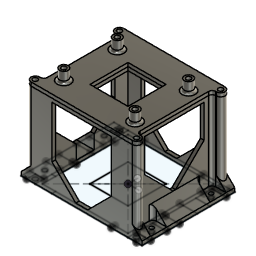
Battery Case (Autodesk Fusion 360 design; units mm, degrees)
Autodesk Fusion 360 part; units mm, degrees
sketch "Sketch1" plane through (0, 0, 0) normal (0, 0, 1) x (1, 0, 0)
  line L0 (36, 36) -> (-36, 36)
  line L1 (-36, 36) -> (-36, -36)
  line L2 (-36, -36) -> (36, -36)
  line L3 (36, -36) -> (36, 36)
  line L4 (36, 36) -> (-36, -36) construction
  line L5 (-36, 36) -> (36, -36) construction
  line L6 (-39, 39) -> (39, 39)
  line L7 (39, 39) -> (39, -39)
  line L8 (39, -39) -> (-39, -39)
  line L9 (-39, -39) -> (-39, 39)
  line L10 (-39, 39) -> (-50.8, 39)
  line L11 (-50.8, 39) -> (-50.8, -39)
  line L12 (-50.8, -39) -> (-39, -39)
  line L13 (39, -39) -> (50.8, -39)
  line L14 (50.8, -39) -> (50.8, 39)
  line L15 (50.8, 39) -> (39, 39)
  circle A0 centre (-45, 25) radius 1.7
  line L16 (0, 0) -> (0, 8)
  line L17 (0, 0) -> (9, 0)
  circle A1 centre (-45, -25) radius 1.7
  circle A2 centre (45, 25) radius 1.7
  circle A3 centre (45, -25) radius 1.7
  line L18 (-39, -25) -> (-36, -25)
  line L19 (39, -25) -> (36, -25)
  line L20 (-39, 25) -> (-36, 25)
  line L21 (39, 25) -> (36, 25)
  line L22 (-25, -39) -> (-25, -36)
  line L23 (25, -39) -> (25, -36)
  line L24 (-25, 39) -> (-25, 36)
  line L25 (25, 39) -> (25, 36)
  line L26 (-50.8, 31.8) -> (-39, 31.8)
  line L27 (50.8, 31.8) -> (39, 31.8)
  line L28 (-50.8, -31.8) -> (-39, -31.8)
  line L29 (50.8, -31.8) -> (39, -31.8)
  circle A4 centre (-42.6, 35.4) radius 2
  line L30 (-39, 31.8) -> (-46.2, 31.8)
  line L31 (-46.2, 31.8) -> (-46.2, 39)
  line L32 (-42.6, 35.4) -> (-39, 35.4)
  line L33 (-42.6, 35.4) -> (-42.6, 31.8)
  line L34 (-42.6, 35.4) -> (-46.2, 35.4)
  line L35 (-42.6, 35.4) -> (-42.6, 39)
  line L36 (39, 31.8) -> (46.2, 31.8)
  line L37 (46.2, 31.8) -> (46.2, 39)
  circle A5 centre (42.6, 35.4) radius 2
  line L38 (39, -31.8) -> (46.2, -31.8)
  line L39 (46.2, -31.8) -> (46.2, -39)
  circle A6 centre (42.6, -35.4) radius 2
  line L40 (-39, -31.8) -> (-46.2, -31.8)
  line L41 (-46.2, -31.8) -> (-46.2, -39)
  circle A7 centre (-42.6, -35.4) radius 2
  line L42 (-16, -16) -> (16, -16)
  line L43 (16, -16) -> (16, 16)
  line L44 (16, 16) -> (-16, 16)
  line L45 (-16, 16) -> (-16, -16)
  line L46 (-16, -16) -> (16, 16) construction
  line L47 (16, -16) -> (-16, 16) construction
  line L48 (-39, 7.5) -> (-36, 7.5)
  line L49 (39, 7.5) -> (36, 7.5)
  line L50 (-39, -7.5) -> (-36, -7.5)
  line L51 (39, -7.5) -> (36, -7.5)
  line L52 (39, 7.5) -> (50.8, 7.5)
  line L53 (50.8, 18.2) -> (39, 18.2)
  line L54 (-39, 7.5) -> (-50.8, 7.5)
  line L55 (-50.8, 18.2) -> (-39, 18.2)
  line L56 (39, -7.5) -> (50.8, -7.5)
  line L57 (50.8, -18.2) -> (39, -18.2)
  line L58 (-39, -7.5) -> (-50.8, -7.5)
  line L59 (-50.8, -18.2) -> (-39, -18.2)
  dimension "d1" = 72
  dimension "d2" = 72
  dimension "d3" = 3
  dimension "d4" = 3
  dimension "d5" = 3
  dimension "d6" = 3
  dimension "d7" = 101.6
  dimension "d8" = 50
  dimension "d9" = 90
  dimension "d10" = 3.4
  dimension "d13" = 50
  dimension "d14" = 50
  dimension "d20" = 7.2
  dimension "d24" = 4
  dimension "d25" = 7.2
  dimension "d27" = 7.2
  dimension "d34" = 20
  dimension "d37" = 15
  dimension "d38" = 6.8
  constraint horizontal L0
  constraint perpendicular L0 L1
  constraint parallel L0 L2
  constraint parallel L1 L3
  constraint coincident L4 L16.start
  constraint coincident L5 L16.start
  constraint coincident L16.start L17.start
  constraint horizontal L6
  constraint vertical L7
  constraint horizontal L8
  constraint vertical L9
  constraint perpendicular L9 L10
  constraint perpendicular L10 L11
  constraint perpendicular L14 L15
  constraint perpendicular L13 L14
  constraint perpendicular L7 L13
  constraint perpendicular L11 L12
  constraint equal L10 L15
  constraint vertical L16
  constraint perpendicular L16 L17
  constraint symmetric A0 L17 A1
  constraint symmetric A0 L16 A2
  constraint symmetric L16 A1 A3
  constraint coincident L9 L18.start
  constraint coincident L1 L18.end
  constraint perpendicular L1 L18
  constraint symmetric L16 L18.start L19.start
  constraint symmetric L16 L18.end L19.end
  constraint symmetric L17 L18.start L20.start
  constraint symmetric L17 L18.end L20.end
  constraint symmetric L17 L19.start L21.start
  constraint symmetric L17 L19.end L21.end
  constraint coincident L8 L22.start
  constraint coincident L2 L22.end
  constraint perpendicular L2 L22
  constraint symmetric L16 L22.start L23.start
  constraint symmetric L16 L22.end L23.end
  constraint symmetric L17 L22.start L24.start
  constraint symmetric L17 L22.end L24.end
  constraint symmetric L17 L23.start L25.start
  constraint symmetric L17 L23.end L25.end
  constraint coincident L11 L26.start
  constraint coincident L9 L26.end
  constraint perpendicular L9 L26
  constraint symmetric L16 L26.start L27.start
  constraint symmetric L16 L26.end L27.end
  constraint symmetric L17 L26.start L28.start
  constraint symmetric L17 L26.end L28.end
  constraint symmetric L17 L27.start L29.start
  constraint symmetric L17 L27.end L29.end
  constraint perpendicular L9 L30
  constraint coincident L10 L31.end
  constraint perpendicular L10 L31
  constraint coincident A4.centre L32.start
  constraint coincident L9 L32.end
  constraint perpendicular L9 L32
  constraint coincident L30 L33.end
  constraint perpendicular L30 L33
  constraint coincident L31 L34.end
  constraint perpendicular L31 L34
  constraint coincident L10 L35.end
  constraint perpendicular L10 L35
  constraint equal L32 L34
  constraint equal L33 L35
  constraint symmetric L16 A4 A5
  constraint symmetric L16 L30.end L36.end
  constraint symmetric L16 L31.end L37.end
  constraint symmetric L17 A4 A7
  constraint symmetric L17 L30.end L40.end
  constraint symmetric L17 L31.end L41.end
  constraint symmetric L17 L36.end L38.end
  constraint symmetric L17 L37.end L39.end
  constraint symmetric L17 A5 A6
  constraint horizontal L42
  constraint perpendicular L42 L43
  constraint parallel L42 L44
  constraint parallel L43 L45
  constraint coincident L46 L16.start
  constraint coincident L47 L16.start
  constraint coincident L4 L42.start
  constraint coincident L9 L48.start
  constraint coincident L1 L48.end
  constraint perpendicular L1 L48
  constraint symmetric L16 L48.start L49.start
  constraint symmetric L16 L48.end L49.end
  constraint symmetric L17 L48.start L50.start
  constraint symmetric L17 L48.end L50.end
  constraint symmetric L17 L49.start L51.start
  constraint symmetric L17 L49.end L51.end
  constraint coincident L14 L52.end
  constraint perpendicular L14 L52
  constraint coincident L14 L53.start
  constraint coincident L7 L53.end
  constraint perpendicular L7 L53
  constraint symmetric L16 L49.start L48.start
  constraint symmetric L16 L52.end L54.end
  constraint symmetric L16 L53.start L55.start
  constraint symmetric L16 L53.end L55.end
  constraint symmetric L17 L52.end L56.end
  constraint symmetric L17 L53.start L57.start
  constraint symmetric L17 L53.end L57.end
  constraint symmetric L17 L54.end L58.end
  constraint symmetric L17 L55.start L59.start
  constraint symmetric L17 L55.end L59.end
  measures "d1" distance of L0.start L0.end
  measures "d2" distance of L0.start L2.end
  measures "d3" distance of L3 L7
  measures "d4" distance of L0 L6
  measures "d5" distance of L1 L9
  measures "d6" distance of L2 L8
  measures "d7" distance of L11 L14
  measures "d8" distance of A0.centre A1.centre
  measures "d9" distance of A0.centre A2.centre
  measures "d10" diameter of A0
  measures "d13" distance of L22 L23
  measures "d14" distance of L18 L20
  measures "d20" distance of L10 L26
  measures "d24" diameter of A4
  measures "d25" distance of L10 L30
  measures "d27" distance of L9 L31
  measures "d34" distance of L3 L43
  measures "d37" distance of L48 L50
  measures "d38" distance of A2.centre L53
extrude "Extrude1" add sketch "Sketch1" along normal blind 3 contours L0 L1 L2 L3 | L0 L3 L6 L7 L21 L25 | L0 L6 L24 L25 | L3 L7 L21 L49 | L0 L1 L6 L9 L20 L24 | L3 L7 L49 L51 | L7 L15 L27 L36 L37 | L3 L7 L19 L51 | L1 L9 L20 L48 | L9 L10 A4 L32 L35 | L2 L3 L7 L8 L19 L23 | L1 L9 L48 L50 | L9 L26 A4 L30 L32 L33 | L10 A4 L31 L34 L35 | L1 L9 L18 L50 | L2 L8 L22 L23 | L7 L13 L29 L38 L39 | L1 L2 L8 L9 L18 L22 | L26 A4 L30 L31 L33 L34 | L9 L12 L28 L40 L41 makes body 1
extrude "Extrude2" add sketch "Sketch1" against normal blind 66.5 contours L0 L3 L6 L7 L21 L25 | L0 L1 L6 L9 L20 L24 | L7 L15 L27 L36 L37 | L9 L10 A4 L32 L35 | L2 L3 L7 L8 L19 L23 | L9 L26 A4 L30 L32 L33 | L10 A4 L31 L34 L35 | A4 L32 L35 | A4 L32 L33 | A4 L34 L35 | L7 L13 L29 L38 L39 | L1 L2 L8 L9 L18 L22 | L26 A4 L30 L31 L33 L34 | A4 L33 L34 | L9 L12 L28 L40 L41 | A5 | A6 | A7 bodies 1
extrude "Extrude5" cut sketch "Sketch1" against normal blind 15 contours A4 L32 L35 | A4 L32 L33 | A4 L34 L35 | A4 L33 L34 | A5 | A6 | A7 bodies 1
fillet "Fillet1" radius 3 4 edges at (39, -31.8, -31.75) (39, 31.8, -31.75) (-39, 31.8, -31.75) (-39, -31.8, -31.75) on bodies 1
move_body "Move1" bodies 1 to x (1, 0, 0) y (0, 1, 0) z (0, 0, 1) at (0, 0, 66.5)
extrude "Extrude3" add sketch "Sketch1" along normal blind 3 contours L0 L3 L6 L7 L21 L25 | L0 L6 L24 L25 | L3 L7 L21 L49 | L0 L1 L6 L9 L20 L24 | L3 L7 L49 L51 | L7 L14 L27 L36 L53 | L7 L15 L27 L36 L37 | L3 L7 L19 L51 | L7 L14 L52 L56 | L7 L14 L52 L53 | L1 L9 L20 L48 | L9 L10 A4 L32 L35 | L14 L15 L27 L37 | L2 L3 L7 L8 L19 L23 | L7 L14 L56 L57 | L1 L9 L48 L50 | L9 L11 L26 L30 L55 | L9 L26 A4 L30 L32 L33 | L10 A4 L31 L34 L35 | L7 L14 L29 L38 L57 | L1 L9 L18 L50 | L9 L11 L54 L55 | L9 L11 L54 L58 | A4 L32 L35 | A4 L32 L33 | L10 L11 L26 L31 | A4 L34 L35 | L2 L8 L22 L23 | L7 L13 L29 L38 L39 | L1 L2 L8 L9 L18 L22 | L9 L11 L58 L59 | L26 A4 L30 L31 L33 L34 | A4 L33 L34 | L13 L14 L29 L39 | L9 L11 L28 L40 L59 | L9 L12 L28 L40 L41 | L11 L12 L28 L41 | A5 | A6 | A7 bodies 1
extrude "Extrude4" add sketch "Sketch1" along normal blind 3.2 contours L7 L15 L27 L36 L37 | L9 L10 A4 L32 L35 | L14 L15 L27 L37 | L9 L26 A4 L30 L32 L33 | L10 A4 L31 L34 L35 | A4 L32 L35 | A4 L32 L33 | L10 L11 L26 L31 | A4 L34 L35 | L7 L13 L29 L38 L39 | L26 A4 L30 L31 L33 L34 | A4 L33 L34 | L13 L14 L29 L39 | L9 L12 L28 L40 L41 | L11 L12 L28 L41 | A5 | A6 | A7 bodies 1
chamfer "Chamfer2" distance 4.6 angle 45 4 edges at (46.2, 35.4, 3.2) (46.2, -35.4, 3.2) (-46.2, 35.4, 3.2) (-46.2, -35.4, 3.2) on bodies 1
extrude "Extrude6" add sketch "Sketch1" along normal blind 14.8 contours L3 L7 L21 L49 | L3 L7 L49 L51 | L3 L7 L19 L51 | L1 L9 L20 L48 | L1 L9 L18 L50 bodies 1
extrude "Extrude7" add sketch "Sketch1" along normal blind 3.2 contours L7 L14 L52 L56 | L7 L14 L52 L53 | L7 L14 L56 L57 | L9 L11 L54 L55 | L9 L11 L58 L59 bodies 1
chamfer "Chamfer3" distance 11.6 angle 45 4 edges at (-39, 12.85, 3.2) (-39, -12.85, 3.2) (39, 0, 3.2) (39, 0, 3.2) on bodies 1
chamfer "Chamfer4" distance 0.2 angle 45 4 edges at (-50.8, -12.85, 3.2) (-50.8, 12.85, 3.2) (50.8, 0, 3.2) (50.8, 0, 3.2) on bodies 1
chamfer "Chamfer1" distance 20 angle 45 4 edges at (25, -37.5, 3) (-25, -37.5, 3) (-25, 37.5, 3) (25, 37.5, 3) on bodies 1
chamfer "Chamfer1" distance 17.4 angle 45 2 edges at (-37.5, 25, 14.8) (-37.5, -25, 14.8) on bodies 1
chamfer "Chamfer1" distance 24 angle 45 2 edges at (37.5, -25, 14.8) (37.5, 25, 14.8) on bodies 1
sketch "Sketch2" plane through (0, 0, 69.5) normal (0, 0, 1) x (-1, 0, 0)
  line L0 (16, 16) -> (16, -16)
  line L1 (16, -16) -> (-16, -16)
  line L2 (-16, -16) -> (-16, 16)
  line L3 (-16, 16) -> (16, 16)
  circle A0 centre (42.6, -35.4) radius 2
  circle A1 centre (-42.6, -35.4) radius 2
  circle A2 centre (-42.6, 35.4) radius 2
  circle A3 centre (42.6, 35.4) radius 2
  line L4 (42, 31.8) -> (46.2, 31.8)
  line L5 (46.2, 31.8) -> (46.2, 39)
  line L6 (46.2, 39) -> (-46.2, 39)
  line L7 (-46.2, 39) -> (-46.2, 31.8)
  line L8 (-46.2, 31.8) -> (-42, 31.8)
  arc A4 (-39, 28.8) -> (-42, 31.8) centre (-42, 28.8) ccw
  line L9 (-39, 28.8) -> (-39, -28.8)
  arc A5 (-42, -31.8) -> (-39, -28.8) centre (-42, -28.8) ccw
  line L10 (-42, -31.8) -> (-46.2, -31.8)
  line L11 (-46.2, -31.8) -> (-46.2, -39)
  line L12 (-46.2, -39) -> (46.2, -39)
  line L13 (46.2, -39) -> (46.2, -31.8)
  line L14 (46.2, -31.8) -> (42, -31.8)
  arc A6 (39, -28.8) -> (42, -31.8) centre (42, -28.8) ccw
  line L15 (39, -28.8) -> (39, 28.8)
  arc A7 (42, 31.8) -> (39, 28.8) centre (42, 28.8) ccw
  line L16 (-39, 39) -> (39, 39)
  line L17 (39, 39) -> (39, -39)
  line L18 (39, -39) -> (-39, -39)
  line L19 (-39, -39) -> (-39, 39)
  line L20 (46.2, -39) -> (39, -39)
  line L21 (46.2, -39) -> (46.2, -31.8)
  line L22 (46.2, -31.8) -> (39, -31.8)
  line L23 (46.2, 39) -> (39, 39)
  line L24 (46.2, 31.8) -> (46.2, 39)
  line L25 (46.2, 31.8) -> (39, 31.8)
  line L26 (-46.2, 39) -> (-39, 39)
  line L27 (-46.2, 39) -> (-46.2, 31.8)
  line L28 (-46.2, 31.8) -> (-39, 31.8)
  line L29 (-46.2, -31.8) -> (-39, -31.8)
  line L30 (-46.2, -39) -> (-39, -39)
  line L31 (-46.2, -31.8) -> (-46.2, -39)
  line L32 (30, 24) -> (-30, 24)
  line L33 (-30, 24) -> (-30, -21)
  line L34 (-30, -21) -> (30, -21)
  line L35 (30, -21) -> (30, 24)
  circle A8 centre (30, 24) radius 2
  circle A9 centre (30, -21) radius 2
  circle A10 centre (-30, -21) radius 2
  circle A11 centre (-30, 24) radius 2
  circle A12 centre (30, 24) radius 3.6
  circle A13 centre (30, -21) radius 3.6
  circle A14 centre (-30, -21) radius 3.6
  circle A15 centre (-30, 24) radius 3.6
  point P0 (0, -21)
  point P1 (0, 24)
  dimension "d48" = 4
  dimension "d49" = 60
  dimension "d50" = 45
  dimension "d51" = 15
  dimension "d52" = 7.2
  constraint horizontal L16
  constraint vertical L17
  constraint horizontal L18
  constraint vertical L19
  constraint coincident L12 L17.end
  constraint coincident L6 L16.start
  constraint coincident L12.end L13.start
  constraint perpendicular L13 L20
  constraint coincident L13.end L14.start
  constraint coincident L17 L22.end
  constraint perpendicular L17 L22
  constraint coincident L5.end L6.start
  constraint coincident L4.end L5.start
  constraint coincident L17 L25.end
  constraint perpendicular L17 L25
  constraint coincident L6.end L7.start
  constraint coincident L7.end L8.start
  constraint coincident L19 L28.end
  constraint perpendicular L19 L28
  constraint coincident L10.end L11.start
  constraint coincident L19 L29.end
  constraint perpendicular L19 L29
  constraint coincident L11.end L12.start
  constraint horizontal L32
  constraint vertical L33
  constraint horizontal L34
  constraint vertical L35
  constraint coincident L32.start L35.end
  constraint coincident L34.end L35.start
  constraint coincident L33.end L34.start
  constraint coincident L32.end L33.start
  constraint equal A8 A9
  constraint equal A9 A10
  constraint equal A10 A11
  constraint midpoint L34 P0
  constraint midpoint L32 P1
  constraint collinear P0 P1 origin
  constraint concentric A8 A12
  constraint concentric A9 A13
  constraint concentric A10 A14
  constraint concentric A11 A15
  constraint equal A12 A13
  constraint equal A13 A14
  constraint equal A12 A15
  measures "d48" diameter of A8
  measures "d49" distance of L33.end L34.end
  measures "d50" distance of L32.start L34.end
  measures "d51" distance of L16 L32
  measures "d52" diameter of A12
extrude "Extrude8" add sketch "Sketch2" along normal blind 3 separate body contours L4 L5 L6 L17 L23 L24 L25 | L6 L9 L12 L15 L16 L17 L18 L19 | L12 L13 L14 L17 L20 L21 L22 | L6 L7 L8 L19 L26 L27 L28 | L10 L11 L12 L19 L29 L30 L31 | L32 L33 A11 A15 | L32 L33 A11 A15 | L32 L33 L34 L35 A12 A13 A14 A15 | L32 L33 A11 | L32 L33 A11 | L32 L35 A8 A12 | L32 L35 A8 A12 | L33 L34 A10 A14 | L33 L34 A10 A14 | L34 L35 A9 A13 | L34 L35 A9 A13 | L33 L34 A10 | L33 L34 A10 makes body 2
fillet "Fillet2" radius 3.6 16 edges at (-46.2, -39, 38.65) (-46.2, -31.8, 38.65) (-46.2, 31.8, 38.65) (-46.2, 39, 38.65) (46.2, 39, 38.65) (46.2, 31.8, 38.65) (46.2, -31.8, 38.65) (46.2, -39, 38.65) (46.2, 39, 71) (46.2, 31.8, 71) (46.2, -31.8, 71) (-46.2, -39, 71) (-46.2, -31.8, 71) (-46.2, 31.8, 71) (-46.2, 39, 71) (46.2, -39, 71) on bodies 1 2
fillet "Fillet3" radius 3 4 edges at (-39, -31.8, 71) (-39, 31.8, 71) (39, 31.8, 71) (39, -31.8, 71) on bodies 2
extrude "Extrude9" add sketch "Sketch2" along normal blind 12 contours L32 L33 A11 A15 | L32 L33 A11 A15 | L32 L35 A8 A12 | L32 L35 A8 A12 | L33 L34 A10 A14 | L33 L34 A10 A14 | L34 L35 A9 A13 | L34 L35 A9 A13 bodies 2
fillet "Fillet4" radius 2 4 edges at (-26.6436, -25.3018, 72.5) (-26.6436, 19.6982, 72.5) (33.3564, 19.6982, 72.5) (33.3564, -25.3018, 72.5) on bodies 2
fillet "Fillet5" radius 3 4 edges at (-39, -18.2, 8.9) (-39, 18.2, 8.9) (39, 18.2, 8.9) (39, -18.2, 8.9) on bodies 1
equation "d33 = ( 7.2 / 2 ) * 1 mm"
